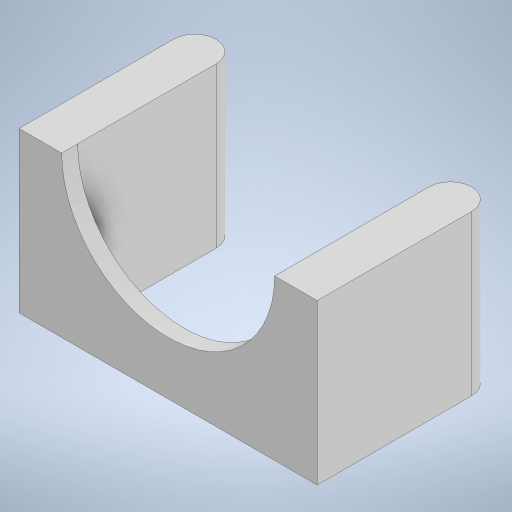
# Autodesk Inventor part: encastre pinza pilar central
Saved by Autodesk Inventor 2024 (Build 280153000, 153)
## iProperties
Created: 2024-05-04
Part Number: encastre pinza pilar central
Material: Generic
Document SubType Name: Modeling
Designer: compu
Density: 1 g/cm^3
Appearance: Default
Author: compu
Autodesk Inventor part; units mm, degrees
ref_plane "YZ Plane" through (0, 0, 0) normal (1, 0, 0) x (0, 1, 0)
ref_plane "XZ Plane" through (0, 0, 0) normal (0, 1, 0) x (-1, 0, 0)
ref_plane "XY Plane" through (0, 0, 0) normal (0, 0, 1) x (1, 0, 0)
sketch "Sketch1" plane through (0, 0, 0) normal (0, 1, 0) x (-1, 0, 0)
  line L0 (14, 0) -> (-14, 0) projected
  line L1 (0, -18.3) -> (0, 4.8) projected
  line L2 (14, 1.5) -> (-14, 1.5)
  line L3 (-14, 1.5) -> (-14, 0)
  line L4 (-10, 0) -> (10, 0)
  line L5 (14, 0) -> (14, 1.5)
  line L6 (10, 0) -> (10, -15)
  line L7 (10, -15) -> (14, -15)
  line L8 (14, -15) -> (14, 0)
  line L9 (-10, 0) -> (-10, -15)
  line L10 (-10, -15) -> (-14, -15)
  line L11 (-14, -15) -> (-14, 0)
  point P0 (0, 0)
  dimension "d0" = 28
  dimension "d1" = 4
  dimension "d2" = 15
  dimension "d3" = 1.5
  dimension "d5" = 4
  dimension "d6" = 15
  constraints: 20 end point, 4 parallel, 2 collinear, 2 point on line, 1 horizontal, 1 perpendicular, 2 other
  measures "d0" distance between parallel lines of L3 L5
  measures "d1" distance of L6.end L7.end
  measures "d2" distance between parallel lines of L0 L7
  measures "d3" distance between parallel lines of L2 L0
  measures "d5" distance of L9.end L10.end
  measures "d6" distance of L10.end L3.end
extrude "Extrusion1" add sketch "Sketch1" along normal blind 15
fillet "Fillet1" radius 2 4 edges at (14, 7.5, -15) (10, 7.5, -15) (-10, 7.5, -15) (-14, 7.5, -15)
sketch "Sketch2" plane through (-14, 0, 1.5) normal (0, 0, 1) x (1, 0, 0)
  line L0 (0, 0) -> (28, 0) projected
  line L1 (28, 0) -> (28, 15) projected
  line L2 (0, 15) -> (28, 15) projected
  line L3 (0, 0) -> (0, 15) projected
  line L4 (24, 0) -> (24, 15) projected
  line L5 (4, 0) -> (4, 15) projected
  circle A0 centre (14, 15) radius 10
  point P0 (14, 0)
  constraints: 1 horizontal alignment, 1 midpoint, 2 other
extrude "Extrusion2" cut sketch "Sketch2" against normal blind 15 contours A0 L2 | L2 A0
body "Solid1"
